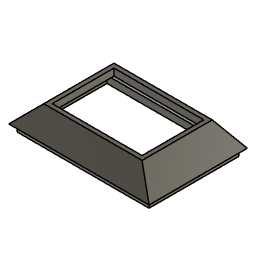
loftpiece v1 (Autodesk Fusion 360 design; units mm, degrees)
Autodesk Fusion 360 part; units mm, degrees
sketch "Sketch1" plane through (0, 0, 0) normal (0, 0, 1) x (1, 0, 0)
  line L0 (0, 0) -> (100, 0)
  line L1 (100, 0) -> (100, -70)
  line L2 (100, -70) -> (0, -70)
  line L3 (0, -70) -> (0, 0)
  line L4 (97, -67) -> (3, -67)
  line L5 (3, -67) -> (3, -3)
  line L6 (3, -3) -> (97, -3)
  line L7 (97, -3) -> (97, -67)
  dimension "d1" = 100
  dimension "d2" = 70
  dimension "d3" = 3
  constraint horizontal L0
  constraint vertical L1
  constraint horizontal L2
  constraint vertical L3
  measures "d1" distance of L0.start L0.end
  measures "d2" distance of L0.start L2.end
ref_plane "WorkPlane1" through (0, 0, 15) normal (0, 0, 1) x (1, 0, 0)
sketch "Sketch2" plane through (0, 0, 15) normal (0, 0, 1) x (1, 0, 0)
  line L0 (15, -10) -> (85, -10)
  line L1 (85, -10) -> (85, -60)
  line L2 (85, -60) -> (15, -60)
  line L3 (15, -60) -> (15, -10)
  line L4 (82, -57) -> (18, -57)
  line L5 (18, -57) -> (18, -13)
  line L6 (18, -13) -> (82, -13)
  line L7 (82, -13) -> (82, -57)
  dimension "d5" = 50
  dimension "d6" = 70
  dimension "d8" = 3
  constraint horizontal L0
  constraint vertical L1
  constraint horizontal L2
  constraint vertical L3
  measures "d5" distance of L0.start L2.end
  measures "d6" distance of L0.start L0.end
loft "Loft1" add profiles "Sketch2", "Sketch1" section 1 section 2
sketch "Sketch3" plane through (0, 0, 15) normal (0, 0, 1) x (-1, 0, 0)
  line L0 (-15, 60) -> (-85, 60)
  line L1 (-85, 60) -> (-85, 10)
  line L2 (-85, 10) -> (-15, 10)
  line L3 (-15, 10) -> (-15, 60)
  line L4 (-18, 57) -> (-82, 57)
  line L5 (-82, 57) -> (-82, 13)
  line L6 (-82, 13) -> (-18, 13)
  line L7 (-18, 13) -> (-18, 57)
  dimension "d10" = -3
extrude "Extrude2" cut sketch "Sketch3" against normal blind 5 contours L4 L5 L6 L7
sketch "Sketch5" plane through (0, 0, 0) normal (0, 0, -1) x (1, 0, 0)
  line L0 (100, 70) -> (0, 70)
  line L1 (0, 70) -> (0, 0)
  line L2 (0, 0) -> (100, 0)
  line L3 (100, 0) -> (100, 70)
  line L4 (5, 5) -> (95, 5)
  line L5 (95, 5) -> (95, 65)
  line L6 (95, 65) -> (5, 65)
  line L7 (5, 65) -> (5, 5)
  dimension "d16" = -5
loft "Loft3" cut profiles "Sketch5" section 1 face at (60.6667, -42.3333, 10) section 2 contours L4 L5 L6 L7
sketch "Sketch6" plane through (0, 0, 0) normal (0, 0, -1) x (1, 0, 0)
  line L0 (95, 5) -> (5, 5)
  line L1 (5, 5) -> (5, 65)
  line L2 (5, 65) -> (95, 65)
  line L3 (95, 65) -> (95, 5)
  line L4 (100, 70) -> (0, 70)
  line L5 (0, 70) -> (0, 0)
  line L6 (0, 0) -> (100, 0)
  line L7 (100, 0) -> (100, 70)
  line L8 (5, 65) -> (95, 65)
  line L9 (95, 65) -> (95, 5)
  line L10 (95, 5) -> (5, 5)
  line L11 (5, 5) -> (5, 65)
  line L12 (97, 3) -> (3, 3)
  line L13 (3, 3) -> (3, 67)
  line L14 (3, 67) -> (97, 67)
  line L15 (97, 67) -> (97, 3)
  dimension "d17" = -2
  constraint horizontal L8
  constraint vertical L9
  constraint horizontal L10
  constraint vertical L11
  constraint coincident L0.start L3.end
  constraint coincident L1.end L2.start
extrude "Extrude3" add sketch "Sketch6" along normal blind 5 contours L12 L13 L14 L15
sketch "Sketch4" plane through (0, 0, 0) normal (0, 0, -1) x (1, 0, 0)
  line L0 (100, 70) -> (0, 70)
  line L1 (0, 70) -> (0, 0)
  line L2 (0, 0) -> (100, 0)
  line L3 (100, 0) -> (100, 70)
  line L4 (5, 5) -> (95, 5)
  line L5 (95, 5) -> (95, 65)
  line L6 (95, 65) -> (5, 65)
  line L7 (5, 65) -> (5, 5)
  dimension "d13" = -5
loft "Loft2" [suppressed]
extrude "Extrude1" [suppressed]
shell "Shell1" [suppressed]
